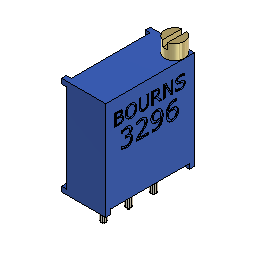
Bourns_3926 (Autodesk Fusion 360 design; units mm, degrees)
Autodesk Fusion 360 part; units mm, degrees
sketch "Sketch1" plane through (0, 0, 0) normal (0, 0, 1) x (1, 0, 0)
  line L0 (5, -4.5) -> (-5, -4.5)
  line L1 (-5, -4.5) -> (-5, 4.5)
  line L2 (-5, 4.5) -> (5, 4.5)
  line L3 (5, 4.5) -> (5, -4.5)
  line L4 (5, -4.5) -> (-5, 4.5) construction
  line L5 (-5, -4.5) -> (5, 4.5) construction
  dimension "d1" = 10
  dimension "d2" = 9
  constraint horizontal L0
  constraint perpendicular L0 L1
  constraint parallel L0 L2
  constraint parallel L1 L3
  constraint coincident L4 origin
  constraint coincident L5 origin
  measures "d1" distance of L1.end L2.end
  measures "d2" distance of L0.end L1.end
extrude "Extrude1" add sketch "Sketch1" along normal blind 4.5 makes body 1
sketch "Sketch2" plane through (5, 0, 0) normal (1, 0, 0) x (0, 1, 0)
  line L0 (-4.5, 0) -> (4.5, 0)
  line L1 (4.5, 0) -> (4.5, 4.5)
  line L2 (4.5, 4.5) -> (-4.5, 4.5)
  line L3 (-4.5, 4.5) -> (-4.5, 0)
  line L4 (-4, 0) -> (4, 0)
  line L5 (4, 0) -> (4, 0.5)
  line L6 (4, 0.5) -> (-4, 0.5)
  line L7 (-4, 0.5) -> (-4, 0)
  dimension "d5" = 0.5
  dimension "d6" = 0.5
  dimension "d7" = 0.5
  constraint horizontal L4
  constraint vertical L5
  constraint horizontal L6
  constraint vertical L7
  constraint coincident L0 L4.start
  measures "d5" distance of L4.start L6.end
  measures "d6" distance of L1 L5
  measures "d7" distance of L3 L7
extrude "Extrude2" cut sketch "Sketch2" against normal blind 10 contours L0 L4 L5 L6 L7 bodies 1
sketch "Sketch3" plane through (0, -4.5, 0) normal (0, -1, 0) x (1, 0, 0)
  line L0 (-5, 0) -> (5, 0)
  line L1 (5, 0) -> (5, 4.5)
  line L2 (5, 4.5) -> (-5, 4.5)
  line L3 (-5, 4.5) -> (-5, 0)
  line L4 (-4.5, 0) -> (4.5, 0)
  line L5 (4.5, 0) -> (4.5, 0.5)
  line L6 (4.5, 0.5) -> (-4.5, 0.5)
  line L7 (-4.5, 0.5) -> (-4.5, 0)
  dimension "d11" = 0.5
  dimension "d12" = 0.5
  dimension "d13" = 0.5
  constraint horizontal L4
  constraint vertical L5
  constraint horizontal L6
  constraint vertical L7
  constraint coincident L0 L4.start
  measures "d11" distance of L4.start L6.end
  measures "d12" distance of L1 L5
  measures "d13" distance of L3 L7
extrude "Extrude3" cut sketch "Sketch3" against normal blind 9 contours L0 L4 L5 L6 L7 bodies 1
sketch "Sketch4" plane through (0, 0, 4.5) normal (0, 0, 1) x (-1, 0, 0)
  line L0 (-5, -4.5) -> (5, -4.5)
  line L1 (5, -4.5) -> (5, 4.5)
  line L2 (5, 4.5) -> (-5, 4.5)
  line L3 (-5, 4.5) -> (-5, -4.5)
  line L4 (5, -4) -> (4.5, -4)
  line L5 (4.5, -4) -> (4.5, 4)
  line L6 (4.5, 4) -> (5, 4)
  line L7 (5, 4) -> (5, -4)
  dimension "d16" = 0.5
  dimension "d17" = 0.5
  dimension "d18" = 0.5
  constraint horizontal L4
  constraint vertical L5
  constraint horizontal L6
  constraint vertical L7
  constraint coincident L1 L4.start
  measures "d16" distance of L4.start L4.end
  measures "d17" distance of L0 L4
  measures "d18" distance of L2 L6
extrude "Extrude4" cut sketch "Sketch4" against normal blind 4 contours L1 L4 L5 L6 L7 bodies 1
sketch "Sketch5" plane through (-4.5, 0, 0) normal (-1, 0, 0) x (0, -1, 0)
  line L0 (4, 4.5) -> (-4, 4.5)
  line L1 (-4, 4.5) -> (-4, 0.5)
  line L2 (-4, 0.5) -> (4, 0.5)
  line L3 (4, 0.5) -> (4, 4.5)
  line L4 (-2.79, 0.5) -> (-2.29, 0.5)
  line L5 (-2.29, 0.5) -> (-2.29, 4.05)
  line L6 (-2.29, 4.05) -> (-2.79, 4.05)
  line L7 (-2.79, 4.05) -> (-2.79, 0.5)
  dimension "d21" = 0.5
  dimension "d23" = 3.55
  dimension "d24" = 1.21
  constraint horizontal L4
  constraint vertical L5
  constraint horizontal L6
  constraint vertical L7
  constraint coincident L2 L4.start
  measures "d21" distance of L4.start L4.end
  measures "d23" distance of L4.start L6.end
  measures "d24" distance of L1 L7
extrude "Extrude5" cut sketch "Sketch5" against normal blind 0.5 contours L2 L4 L5 L6 L7 bodies 1
pattern_linear "R-Pattern1" count 3 spacing 2.54 along (0, -1, 0) of "Extrude5"
sketch "Sketch6" plane through (0, 0, 4.5) normal (0, 0, 1) x (-1, 0, 0)
  line L0 (4.5, 4) -> (5, 4)
  line L1 (5, 4) -> (5, 4.5)
  line L2 (5, 4.5) -> (-5, 4.5)
  line L3 (-5, 4.5) -> (-5, -4.5)
  line L4 (-5, -4.5) -> (5, -4.5)
  line L5 (5, -4.5) -> (5, -4)
  line L6 (5, -4) -> (4.5, -4)
  line L7 (4.5, -4) -> (4.5, 4)
  line L8 (-1.9526, -3.5509) -> (-1.9526, 3.4896) construction
  line L9 (-1.9526, 3.4896) -> (-4.2478, 3.4896) construction
  line L10 (-4.2478, 3.4896) -> (-4.2478, -3.5509) construction
  line L11 (-4.2478, -3.5509) -> (-1.9526, -3.5509) construction
  line L12 (0.1387, -3.547) -> (0.1387, 3.4935) construction
  line L13 (0.1387, 3.4935) -> (-2.1565, 3.4935) construction
  line L14 (-2.1565, 3.4935) -> (-2.1565, -3.547) construction
  line L15 (-2.1565, -3.547) -> (0.1387, -3.547) construction
  dimension "d31" = 1.25
  dimension "d32" = 1.75
  text T0 "BOURNS" font "Verdana" height 1.25 align centre middle in box 7.0405 x 2.2952 at (-1.9526, -3.5509) x (0, 1) y (-1, 0) spacing 1
  text T1 "3296" font "Verdana" height 1.75 align centre middle in box 7.0405 x 2.2952 at (0.1387, -3.547) x (0, 1) y (-1, 0) spacing 1
extrude "Extrude6" cut sketch "Sketch6" against normal blind 0.1 text T0 T1 bodies 1
sketch "Sketch7" plane through (5, 0, 0) normal (1, 0, 0) x (0, 1, 0)
  line L0 (4, 0.5) -> (4, 0)
  line L1 (4, 0) -> (4.5, 0)
  line L2 (4.5, 0) -> (4.5, 4.5)
  line L3 (4.5, 4.5) -> (-4.5, 4.5)
  line L4 (-4.5, 4.5) -> (-4.5, 0)
  line L5 (-4.5, 0) -> (-4, 0)
  line L6 (-4, 0) -> (-4, 0.5)
  line L7 (-4, 0.5) -> (4, 0.5)
  circle A0 centre (-3.5, 3.5) radius 1
  dimension "d35" = 2
  dimension "d52" = 1
  dimension "d53" = 1
  measures "d35" diameter of A0
  measures "d52" distance of L4 A0.centre
  measures "d53" distance of L3 A0.centre
extrude "Extrude7" add sketch "Sketch7" along normal blind 1.5 contours A0 bodies 1
sketch "Sketch8" plane through (6.5, 0, 0) normal (1, 0, 0) x (0, 1, 0)
  circle A0 centre (-3.5, 3.5) radius 1
  line L0 (-4.4682, 3.75) -> (-2.5318, 3.75)
  line L1 (-4.4682, 3.25) -> (-2.5318, 3.25)
  point P0 (-3.5, 3.5)
  dimension "d38" = 0.5
  dimension "d39" = 0.25
  constraint coincident A0 L0.start
  constraint coincident A0 L0.end
  constraint horizontal L0
  constraint coincident A0 L1.start
  constraint coincident A0 L1.end
  constraint parallel L0 L1
  constraint coincident P0 A0.centre
  measures "d38" distance of L0 L1
  measures "d39" distance of L0 P0
extrude "Extrude8" cut sketch "Sketch8" against normal blind 0.65 contours A0 L0 L1 bodies 1
sketch "Sketch9" plane through (-4, 0, 0) normal (-1, 0, 0) x (0, -1, 0)
  line L0 (-2.79, 4.05) -> (-2.79, 0.5)
  line L1 (-2.79, 0.5) -> (-2.29, 0.5)
  line L2 (-2.29, 0.5) -> (-2.29, 4.05)
  line L3 (-2.29, 4.05) -> (-2.79, 4.05)
  line L4 (-2.79, 2.55) -> (-2.29, 2.55)
  line L5 (-2.29, 2.55) -> (-2.29, 2.05)
  line L6 (-2.29, 2.05) -> (-2.79, 2.05)
  line L7 (-2.79, 2.05) -> (-2.79, 2.55)
  dimension "d42" = 0.5
  dimension "d43" = 1.5
  constraint horizontal L4
  constraint vertical L5
  constraint horizontal L6
  constraint vertical L7
  constraint coincident L2 L5.end
  constraint coincident L0 L4.start
  measures "d42" distance of L4.start L6.end
  measures "d43" distance of L3 L4
extrude "Extrude9" add sketch "Sketch9" along normal blind 3.5 separate body contours L0 L2 L4 L5 L6 L7 makes body 2
fillet "Fillet1" radius 0.15 8 edges at (-5.75, 2.79, 2.55) (-5.75, 2.79, 2.05) (-5.75, 2.29, 2.55) (-5.75, 2.29, 2.05) (-7.5, 2.54, 2.55) (-7.5, 2.79, 2.3) (-7.5, 2.29, 2.3) (-7.5, 2.54, 2.05) on bodies 2
pattern_linear "R-Pattern2" count 3 spacing 2.54 along (0, -1, 0) of "Extrude9", "Fillet1" makes body 3 at (-6.2333, -0.2179, 2.1073) makes body 4 at (-5.1167, -2.6471, 2.0502)
combine "Combine1" operation add target body 1 tool bodies 2 3 4
move_body "Move1" bodies 1 to x (-1, 0, 0) y (0, -1, 0) z (0, 0, 1) at (0, 0, 0)
move_body "Move2" bodies 1 to x (0, 0, -1) y (0, 1, 0) z (1, 0, 0) at (0, 0, 0)
move_body "Move3" bodies 1 to x (1, 0, 0) y (0, 1, 0) z (0, 0, 1) at (-2.3, 0, 5)
equation "d24 = 0.93 mm + 0.28 mm"
named bodies: "Bourns_3926"
